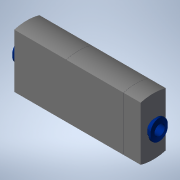
# Autodesk Inventor part: 532624 VN-05-M-I3-PQ2-VQ2-A
Saved by Autodesk Inventor 2021 (Build 250183000, 183)
## iProperties
Created: 2026-04-20
Part Number: 532624 VN-05-M-I3-PQ2-VQ2-A
Material: Generic
Catalog Web Link: www.3dfindit.com
Description: VN2-vacuum generator
Vendor: FESTO
Document SubType Name: Modeling
Designer: psAdmin
Manufacturer: FESTO
Mass: 38 g
Surface Area: 83.8997 cm^2
Volume: 34.3865 cm^3
Density: 1 g/cm^3
Appearance: PSOLRGB-176-176-176
Category: PARTsolutions
Company: FESTO
Title: 532624 VN-05-M-I3-PQ2-VQ2-A
Author: Cadenas PARTsolutions
Comments: vacuum generator
PSOL_IDENT_0: {$CADENAS_DATA/23d-libs/festo/parts/v/vn/vn_2.prj},191 {VTYP=3D},{NB=532624 VN-05-M-I3-PQ2-VQ2-A},{L
PSOL_IDENT_1: INA=532624 VN-05-M-I3-PQ2-VQ2-A},{NN=VN2},{DATE=04.11.2025 07:59:01},{GEOMDATE=04.11.2025 07:59:01},
PSOL_IDENT_2: {VERSION=},{LINEID=70},{WBVAR=},{WBNUMERIC=}  {NB=532624 VN-05-M-I3-PQ2-VQ2-A},{LINA=532624 VN-05-M-
PSOL_IDENT_3: I3-PQ2-VQ2-A},{KT=DUMMY},{TNR=532624},{TYP=VN-05-M-I3-PQ2-VQ2-A},{VERS=11.000},{CNSMASSEXACT=0.038},
PSOL_IDENT_4: {GTIN=4052568086169}
NB: 532624 VN-05-M-I3-PQ2-VQ2-A
NN: VN2
NT: vacuum generator
NBSYN: $TNR. $TYP.
LINA: 532624 VN-05-M-I3-PQ2-VQ2-A
CATALOG: Festo
TNR: 532624
TYP: VN-05-M-I3-PQ2-VQ2-A
CNSMASSEXACT: 0.038
GTIN: 4052568086169
SUPPLIER: FESTO
ARTICLENO: 532624 VN-05-M-I3-PQ2-VQ2-A
BOMINFO: 532624 VN-05-M-I3-PQ2-VQ2-A
CREATOR: CADENAS GmbH
Autodesk Inventor part; units mm, degrees
ref_plane "YZ Plane" through (0, 0, 0) normal (1, 0, 0) x (0, 1, 0)
ref_plane "XZ Plane" through (0, 0, 0) normal (0, 1, 0) x (-1, 0, 0)
ref_plane "XY Plane" through (0, 0, 0) normal (0, 0, 1) x (1, 0, 0)
sketch "Sketch_1" plane through (0, 0, 0) normal (1, 0, 0) x (0, 1, 0)
  arc A0 (-15.55, 7.25) -> (-15.55, -7.25) centre (10.2312, 0) ccw
  line L0 (-15.55, -7.25) -> (15.55, -7.25)
  arc A1 (15.55, -7.25) -> (15.55, 7.25) centre (-10.2312, 0) ccw
  line L1 (15.55, 7.25) -> (-15.55, 7.25)
  constraints: 4 end point, 4 point on circle, 2 centre point
extrude "Extrusion1" add sketch "Sketch_1" along normal blind 73
sketch "Sketch_8" plane through (0, 0, 0) normal (0, 0, 1) x (1, 0, 0)
  line L0 (0, 0) -> (-3.8, 0)
  line L1 (-3.8, 0) -> (-3.8, 3)
  line L2 (-3.8, 3) -> (-3.271, 6)
  line L3 (-3.271, 6) -> (-2.15, 6)
  line L4 (-2.15, 6) -> (-2.15, 4.36)
  line L5 (-2.15, 4.36) -> (-0.65, 4.36)
  line L6 (-0.65, 4.36) -> (-0.65, 3.4)
  line L7 (-0.65, 3.4) -> (0, 3.4)
  line L8 (0, 3.4) -> (0, 0)
  line L9 (0, 0) -> (-3.8, 0)
  constraints: 20 end point
revolve "Revolution1" add sketch "Sketch_8" angle 360 about axis through (0, 0, 0) along (1, 0, 0)
sketch "Sketch_2" plane through (0, 0, 0) normal (0, 0, 1) x (1, 0, 0)
  line L0 (4.2, 0) -> (-3.95, 0)
  line L1 (-3.95, 0) -> (-3.95, 3.15)
  line L2 (-3.95, 3.15) -> (-3.8, 3.15)
  arc A0 (-3.8, 3.15) -> (-3.65, 3) centre (-3.65, 3.15) ccw
  line L3 (-3.65, 3) -> (4.2, 3)
  line L4 (4.2, 3) -> (4.2, 0)
  line L5 (4.2, 0) -> (-3.95, 0)
  constraints: 12 end point, 2 point on circle, 1 centre point
revolve "Revolution2" cut sketch "Sketch_2" angle 360 about axis through (4.2, 0, 0) along (1, 0, 0)
sketch "Sketch_9" plane through (-3.8, 0, 0) normal (1, 0, 0) x (0, 0, -1)
  circle A0 centre (0, 0) radius 7
  arc A1 (-4.9, -0.975) -> (4.9, -0.975) centre (0, -0.975) ccw
  line L0 (4.9, -0.975) -> (4.9, 0.975)
  arc A2 (4.9, 0.975) -> (-4.9, 0.975) centre (0, 0.975) ccw
  line L1 (-4.9, 0.975) -> (-4.9, -0.975)
  constraints: 4 end point, 4 point on circle, 3 centre point
extrude "Extrusion2" cut sketch "Sketch_9" along normal blind 1.65
sketch "Sketch_10" plane through (-2.15, 0, 0) normal (1, 0, 0) x (0, 1, 0)
  circle A0 centre (0, 0) radius 6
  arc A1 (1.4185, -4.1228) -> (-1.4185, -4.1228) centre (0, 0) ccw
  arc A2 (-1.4185, -4.1228) -> (-1.2558, -4.15) centre (-1.2558, -3.65) ccw
  line L0 (-1.2558, -4.15) -> (1.2558, -4.15)
  arc A3 (1.2558, -4.15) -> (1.4185, -4.1228) centre (1.2558, -3.65) ccw
  constraints: 6 point on circle, 4 centre point, 2 end point
extrude "Extrusion3" cut sketch "Sketch_10" along normal blind 1.5
sketch "Sketch_3" plane through (0, 0, 0) normal (0, 0, 1) x (1, 0, 0)
  line L0 (76.8, 0) -> (73, 0)
  line L1 (73, 0) -> (73, 3.4)
  line L2 (73, 3.4) -> (73.65, 3.4)
  line L3 (73.65, 3.4) -> (73.65, 4.36)
  line L4 (73.65, 4.36) -> (75.15, 4.36)
  line L5 (75.15, 4.36) -> (75.15, 6)
  line L6 (75.15, 6) -> (76.271, 6)
  line L7 (76.271, 6) -> (76.8, 3)
  line L8 (76.8, 3) -> (76.8, 0)
  line L9 (76.8, 0) -> (73, 0)
  constraints: 20 end point
revolve "Revolution3" add sketch "Sketch_3" angle 360 about axis through (76.8, 0, 0) along (1, 0, 0)
sketch "Sketch_4" plane through (0, 0, 0) normal (0, 0, 1) x (1, 0, 0)
  line L0 (76.95, 0) -> (68.8, 0)
  line L1 (68.8, 0) -> (68.8, 3)
  line L2 (68.8, 3) -> (76.65, 3)
  arc A0 (76.65, 3) -> (76.8, 3.15) centre (76.65, 3.15) ccw
  line L3 (76.8, 3.15) -> (76.95, 3.15)
  line L4 (76.95, 3.15) -> (76.95, 0)
  line L5 (76.95, 0) -> (68.8, 0)
  constraints: 12 end point, 2 point on circle, 1 centre point
revolve "Revolution4" cut sketch "Sketch_4" angle 360 about axis through (76.95, 0, 0) along (1, 0, 0)
sketch "Sketch_5" plane through (76.8, 0, 0) normal (1, 0, 0) x (0, 0, -1)
  circle A0 centre (0, 0) radius 7
  arc A1 (-4.9, -0.975) -> (4.9, -0.975) centre (0, -0.975) ccw
  line L0 (4.9, -0.975) -> (4.9, 0.975)
  arc A2 (4.9, 0.975) -> (-4.9, 0.975) centre (0, 0.975) ccw
  line L1 (-4.9, 0.975) -> (-4.9, -0.975)
  constraints: 4 end point, 4 point on circle, 3 centre point
extrude "Extrusion4" cut sketch "Sketch_5" against normal blind 1.65
sketch "Sketch_11" plane through (75.15, 0, 0) normal (-1, 0, 0) x (0, 1, 0)
  circle A0 centre (0, 0) radius 6
  arc A1 (1.4185, -4.1228) -> (-1.4185, -4.1228) centre (0, 0) ccw
  arc A2 (-1.4185, -4.1228) -> (-1.2558, -4.15) centre (-1.2558, -3.65) ccw
  line L0 (-1.2558, -4.15) -> (1.2558, -4.15)
  arc A3 (1.2558, -4.15) -> (1.4185, -4.1228) centre (1.2558, -3.65) ccw
  constraints: 6 point on circle, 4 centre point, 2 end point
extrude "Extrusion5" cut sketch "Sketch_11" along normal blind 1.5
sketch "Sketch_6" plane through (30, 0, 0) normal (1, 0, 0) x (0, 0, -1)
  line L0 (-10, -20) -> (10, -20)
  line L1 (10, -20) -> (10, 20)
  line L2 (10, 20) -> (-10, 20)
  line L3 (-10, 20) -> (-10, -20)
  arc A0 (-7.15, -15.45) -> (7.15, -15.45) centre (0, 9.6112) ccw
  line L4 (7.15, -15.45) -> (7.15, 15.45)
  arc A1 (7.15, 15.45) -> (-7.15, 15.45) centre (0, -9.6112) ccw
  line L5 (-7.15, 15.45) -> (-7.15, -15.45)
  constraints: 12 end point, 4 point on circle, 2 centre point
extrude "Extrusion6" cut sketch "Sketch_6" along normal blind 0.1
sketch "Sketch_7" plane through (63, 0, 0) normal (1, 0, 0) x (0, 0, -1)
  line L0 (-10, -20) -> (10, -20)
  line L1 (10, -20) -> (10, 20)
  line L2 (10, 20) -> (-10, 20)
  line L3 (-10, 20) -> (-10, -20)
  arc A0 (-7.15, -15.45) -> (7.15, -15.45) centre (0, 9.6112) ccw
  line L4 (7.15, -15.45) -> (7.15, 15.45)
  arc A1 (7.15, 15.45) -> (-7.15, 15.45) centre (0, -9.6112) ccw
  line L5 (-7.15, 15.45) -> (-7.15, -15.45)
  constraints: 12 end point, 4 point on circle, 2 centre point
extrude "Extrusion7" cut sketch "Sketch_7" along normal blind 0.1
body "Solid1"
